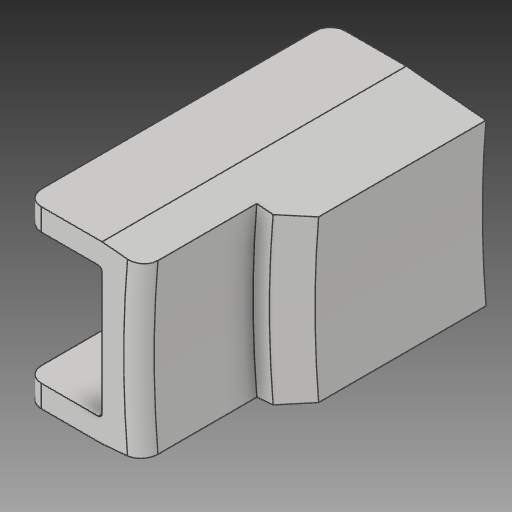
# Autodesk Inventor part: accesorios separador 1
Saved by Autodesk Inventor 2019 (Build 230136000, 136)
## iProperties
Created: 2020-06-11
Part Number: accesorios separador 1
Material: Generic
Document SubType Name: Modeling
Designer: Hugo Albarracin
Density: 1 g/cm^3
Appearance: Default
Author: Hugo Albarracin
Autodesk Inventor part; units mm, degrees
ref_plane "YZ Plane" through (0, 0, 0) normal (1, 0, 0) x (0, 1, 0)
ref_plane "XZ Plane" through (0, 0, 0) normal (0, 1, 0) x (-1, 0, 0)
ref_plane "XY Plane" through (0, 0, 0) normal (0, 0, 1) x (1, 0, 0)
sketch "Sketch1" plane through (0, 0, 0) normal (0, 0, 1) x (1, 0, 0)
  arc A0 (-118.3794, 10.5655) -> (-118.3794, -10.5655) centre (0, 0) ccw
  line L0 (0, 0) -> (-118.85, 0) construction
  line L1 (0, 0) -> (-118.3794, -10.5655) construction
  line L2 (-118.3794, -10.5655) -> (-118.3794, 0) construction
  line L3 (-128.85, 11.5) -> (-118.3794, 10.5655)
  line L4 (-118.3794, 0) -> (-118.3794, 10.5655) construction
  arc A1 (-128.85, 11.5) -> (-128.85, -11.5) centre (0, 0) ccw construction
  line L5 (-118.3794, 10.5655) -> (0, 0) construction
  line L6 (-118.3794, -10.5655) -> (-128.85, -11.5)
  arc A2 (-118.3794, -10.5655) -> (-118.3794, 10.5655) centre (0, 0) ccw construction
  arc A3 (-128.85, -11.5) -> (-128.85, 11.5) centre (0, 0) ccw construction
  line L7 (-128.85, 11.5) -> (-128.85, -11.5)
  dimension "d0" = 237.7
  dimension "d33" = 23
  dimension "d34" = 128.85
  dimension "d37" = 10
  constraints: 16 end point, 9 point on circle, 4 centre point, 3 vertical, 2 coincident, 2 collinear, 1 horizontal, 1 point on line
  measures "d0" diameter of A0
  measures "d33" distance of L3.start L6.end
  measures "d34" distance from line of L7 point (0, 0)
  measures "d37" distance from line of L0.end L7
extrude "Extrusion1" add sketch "Sketch1" along normal mid plane 25
chamfer "Chamfer1" distance 3 angle 45 1 edges at (-118.85, 0, 12.5)
sketch "Sketch4" plane through (0, 0, 0) normal (0, 0, 1) x (1, 0, 0)
  line L0 (0, 0) -> (-126.7631, 7.7532) construction
  line L1 (0, 0) -> (-127, 0) construction
  line L2 (0, 0) -> (-126.7631, -7.7532) construction
  arc A0 (-128.85, 11.5) -> (-128.85, -11.5) centre (0, 0) ccw projected
  arc A1 (-121.3676, 10.8322) -> (-121.3676, -10.8322) centre (0, 0) ccw projected
  line L3 (-121.3676, 10.8322) -> (-128.85, 11.5) projected
  line L4 (-128.85, -11.5) -> (-121.3676, -10.8322) projected
  circle A2 centre (0, 0) radius 127 construction
  line L5 (-128.85, 11.5) -> (-128.85, -11.5) projected
  dimension "d25" = 3.5
  dimension "d26" = 3.5
  constraints: 6 end point, 3 point on circle, 1 centre point, 1 coincident, 1 horizontal, 1 other
  measures "d25" angle of L0 L1
  measures "d26" angle of L1 L2
sketch "Sketch7" plane through (0, 0, 12.5) normal (0, 0, 1) x (1, 0, 0)
  arc A0 (-121.3676, 10.8322) -> (-121.3676, -10.8322) centre (0, 0) ccw projected
  line L0 (-121.3676, 10.8322) -> (-128.85, 11.5) projected
  line L1 (-128.85, 11.5) -> (-128.85, -11.5) projected
  line L2 (-128.85, -11.5) -> (-121.3676, -10.8322) projected
  arc A1 (-123.5091, 11.0233) -> (-123.5091, -11.0233) centre (0, 0) ccw
  arc A2 (-123.5091, -11.0233) -> (-123.5091, 11.0233) centre (0, 0) ccw construction
  line L3 (-128.85, 11.5) -> (-123.5091, 11.0233)
  line L4 (-128.85, -11.5) -> (-123.5091, -11.0233)
  line L5 (-128.85, 11.4972) -> (-128.85, -11.5)
  dimension "d44" = 248
  constraints: 6 end point, 4 point on circle, 3 point on line, 2 centre point, 2 collinear, 1 coincident
  measures "d44" diameter of A1
extrude "Extrusion8" add sketch "Sketch7" along normal blind 15 contours A1 L2 L1 L0
sketch "Sketch8" plane through (-128.85, -11.5, -12.5) normal (-1, 0, 0) x (0, 0, 1)
  line L0 (0, 0) -> (0, 23) projected
  line L1 (40, 23) -> (40, 0) projected
  line L2 (0, 23) -> (40, 23)
  line L3 (40, 23) -> (40, 20.1)
  line L4 (40, 20.1) -> (0, 20.1)
  line L5 (0, 20.1) -> (0, 23)
  line L6 (0, 0) -> (40, 0)
  line L7 (40, 0) -> (40, 2.9)
  line L8 (40, 2.9) -> (0, 2.9)
  line L9 (0, 2.9) -> (0, 0)
  dimension "d48" = 2.9
  dimension "d49" = 2.9
  constraints: 16 end point, 4 parallel, 2 horizontal, 2 perpendicular, 2 point on line
  measures "d48" distance between parallel lines of L4 L2
  measures "d49" distance between parallel lines of L6 L8
extrude "Extrusion7" add sketch "Sketch8" along normal blind 10 contours L0 L8 L1 L6 | L0 L2 L1 L4
fillet "Fillet3" radius 0.5 2 edges at (-128.85, 8.6, 7.5) (-128.85, -8.6, 7.5)
fillet "Fillet4" radius 2 5 edges at (-138.85, 10.05, 27.5) (-138.85, -10.05, 27.5) (-138.85, 10.05, -12.5) (-138.85, -10.05, -12.5) (-124, 0, 27.5)
equation "\"d26\" = d25"
equation "\"d44\" = diametro_max_soporte"
equation "\"d49\" = d48"
equation "\"angulo_alabe\" = 130deg"
equation "\"diametro_tubo\" = 232"
equation "\"desfase_a_pin_superior\" = 12"
equation "\"desfase_b_pin_inferior\" = 8"
equation "\"desfase_b_pin_superior\" = 0"
equation "\"diametro_max_soporte\" = 248"
body "Solid1"
